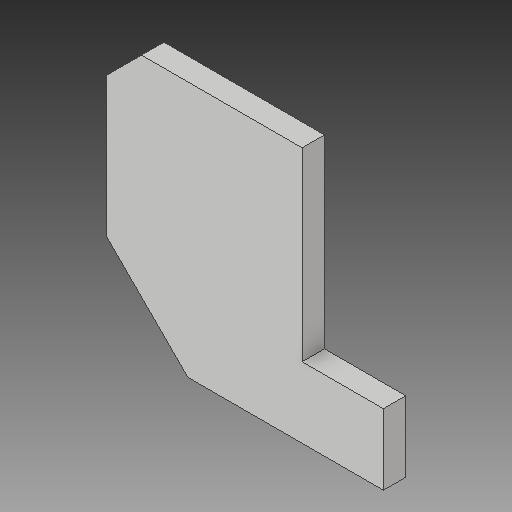
# Autodesk Inventor part: SUPORTE_MANCAL_FRONTAL
Saved by Autodesk Inventor 2018 (Build 220112000, 112)
## iProperties
Created: 2018-10-24
Part Number: SUPORTE_MANCAL_FRONTAL
Material: Genérico
Document SubType Name: Modeling
Designer: Georgines
Density: 1 g/cm^3
Appearance: Padrão
Author: Georgines
Autodesk Inventor part; units mm, degrees
ref_plane "YZ Plane" through (0, 0, 0) normal (1, 0, 0) x (0, 1, 0)
ref_plane "XZ Plane" through (0, 0, 0) normal (0, 1, 0) x (-1, 0, 0)
ref_plane "XY Plane" through (0, 0, 0) normal (0, 0, 1) x (1, 0, 0)
sketch "Esboço1" plane through (0, 0, 0) normal (0, 0, 1) x (1, 0, 0)
  line L0 (-70.9188, 104.3152) -> (40.0812, 104.3152)
  line L1 (-70.9188, 5.5999) -> (-70.9188, 104.3152)
  line L2 (-24.6341, -40.6848) -> (86.1475, -40.6848)
  line L3 (86.1475, -40.6848) -> (86.1475, -0.6848)
  line L4 (86.1475, -0.6848) -> (40.0812, -0.6848)
  line L5 (40.0812, -0.6848) -> (40.0812, 104.3152)
  line L6 (-24.6341, -40.6848) -> (-70.9188, 5.5999)
  line L7 (-24.6341, -40.6848) -> (40.8222, -40.6848) construction
  point P0 (0, 0)
  dimension "d0" = 111
  dimension "d5" = 40
  dimension "d6" = 105
  dimension "d7" = 135
  dimension "d8" = 98.7154
  dimension "d11" = 157.0662
  constraints: 16 end point, 4 horizontal, 2 perpendicular, 1 equal length, 1 parallel
  measures "d0" distance of L0.start L0.end
  measures "d5" distance of L2.end L3.end
  measures "d6" distance of L4.end L0.end
  measures "d7" angle of L7 L6
  measures "d8" distance of L1.start L0.start
  measures "d11" distance between parallel lines of L1 L3
extrude "Extrusão1" add sketch "Esboço1" along normal blind 12.7
chamfer "Chanfro1" distance 20 angle 45 1 edges at (-70.9188, 104.3152, 6.35)
